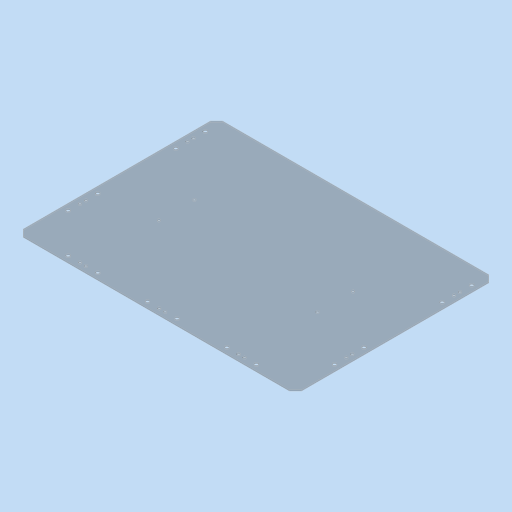
# Autodesk Inventor part: enc-SidePanel Unten 500x708
Saved by Autodesk Inventor 2023.2 (Build 272271000, 271)
## iProperties
Created: 2023-11-30
Part Number: enc-SidePanel Unten 500x708
Material: Generisch
Document SubType Name: Modeling
Designer: Nils Bade
Density: 1 g/cm^3
Appearance: PVC Verglasung
Author: Nils Bade
Autodesk Inventor part; units mm, degrees
ref_plane "YZ Plane" through (0, 0, 0) normal (1, 0, 0) x (0, 1, 0)
ref_plane "XZ Plane" through (0, 0, 0) normal (0, 1, 0) x (-1, 0, 0)
ref_plane "XY Plane" through (0, 0, 0) normal (0, 0, 1) x (1, 0, 0)
sketch "Skizze1" plane through (0, 0, 0) normal (0, 1, 0) x (-1, 0, 0)
  line L0 (0, 0) -> (-698, 0)
  line L1 (-698, 0) -> (-698, 500)
  line L2 (-698, 500) -> (0, 500)
  line L3 (0, 500) -> (0, 0)
  line L4 (-349, 0) -> (-349, 500) construction
  line L5 (0, 250) -> (-698, 250) construction
  line L6 (-150, 0) -> (-150, 500) construction
  line L7 (-548, 0) -> (-548, 500) construction
  line L8 (-698, 350) -> (0, 350) construction
  line L9 (0, 80) -> (-698, 80) construction
  line L10 (-683, 485) -> (-683, 15) construction
  line L11 (-683, 15) -> (-15, 15) construction
  line L12 (-15, 15) -> (-15, 485) construction
  line L13 (-15, 485) -> (-683, 485) construction
  line L14 (-23, 302.5) -> (-7, 302.5) construction
  line L15 (-7, 302.5) -> (-7, 397.5) construction
  line L16 (-7, 397.5) -> (-23, 397.5) construction
  line L17 (-23, 397.5) -> (-23, 302.5) construction
  line L18 (-23, 302.5) -> (-7, 397.5) construction
  line L19 (-7, 302.5) -> (-23, 397.5) construction
  line L20 (-102.5, 493) -> (-197.5, 493) construction
  line L21 (-197.5, 493) -> (-197.5, 477) construction
  line L22 (-197.5, 477) -> (-102.5, 477) construction
  line L23 (-102.5, 477) -> (-102.5, 493) construction
  line L24 (-102.5, 493) -> (-197.5, 477) construction
  line L25 (-197.5, 493) -> (-102.5, 477) construction
  line L26 (-301.5, 493) -> (-396.5, 493) construction
  line L27 (-396.5, 493) -> (-396.5, 477) construction
  line L28 (-396.5, 477) -> (-301.5, 477) construction
  line L29 (-301.5, 477) -> (-301.5, 493) construction
  line L30 (-301.5, 493) -> (-396.5, 477) construction
  line L31 (-396.5, 493) -> (-301.5, 477) construction
  circle A0 centre (-15, 342.5) radius 3.25
  circle A1 centre (-15, 313) radius 4.5
  circle A2 centre (-15, 357.5) radius 3.25
  circle A3 centre (-15, 387) radius 4.5
  circle A4 centre (-142.5, 485) radius 3.25
  circle A5 centre (-113, 485) radius 4.5
  circle A6 centre (-312, 485) radius 4.5
  circle A7 centre (-341.5, 485) radius 3.25
  circle A8 centre (-157.5, 485) radius 3.25
  circle A9 centre (-187, 485) radius 4.5
  circle A10 centre (-386, 485) radius 4.5
  circle A11 centre (-356.5, 485) radius 3.25
  circle A12 centre (-683, 342.5) radius 3.25
  circle A13 centre (-683, 313) radius 4.5
  circle A14 centre (-683, 387) radius 4.5
  circle A15 centre (-683, 357.5) radius 3.25
  circle A16 centre (-555.5, 485) radius 3.25
  circle A17 centre (-585, 485) radius 4.5
  circle A18 centre (-540.5, 485) radius 3.25
  circle A19 centre (-511, 485) radius 4.5
  circle A20 centre (-15, 43) radius 4.5
  circle A21 centre (-15, 72.5) radius 3.25
  circle A22 centre (-150, 205.5) radius 3.25
  line L32 (-138.5, 196) -> (-161.5, 196) construction
  line L33 (-161.5, 196) -> (-161.5, 304) construction
  line L34 (-161.5, 304) -> (-138.5, 304) construction
  line L35 (-138.5, 304) -> (-138.5, 196) construction
  line L36 (-138.5, 196) -> (-161.5, 304) construction
  line L37 (-161.5, 196) -> (-138.5, 304) construction
  circle A23 centre (-150, 294.5) radius 3.25
  circle A24 centre (-548, 205.5) radius 3.25
  circle A25 centre (-548, 294.5) radius 3.25
  circle A26 centre (-15, 117) radius 4.5
  circle A27 centre (-15, 87.5) radius 3.25
  circle A28 centre (-683, 43) radius 4.5
  circle A29 centre (-683, 72.5) radius 3.25
  circle A30 centre (-683, 87.5) radius 3.25
  circle A31 centre (-683, 117) radius 4.5
  point P0 (-15, 350)
  point P1 (-150, 485)
  point P2 (-349, 485)
  point P3 (-150, 250)
  dimension "d0" = 698
  dimension "d1" = 500
  dimension "d2" = 150
  dimension "d3" = 80
  dimension "d4" = 150
  dimension "d5" = 150
  dimension "d6" = 15
  dimension "d7" = 16
  dimension "d8" = 95
  dimension "d9" = 95
  dimension "d10" = 16
  dimension "d11" = 95
  dimension "d12" = 16
  dimension "d13" = 6.5
  dimension "d14" = 7.5
  dimension "d15" = 9
  dimension "d16" = 37
  dimension "d17" = 6.5
  dimension "d18" = 9
  dimension "d19" = 7.5
  dimension "d20" = 37
  dimension "d21" = 6.5
  dimension "d22" = 9
  dimension "d23" = 7.5
  dimension "d24" = 37
  dimension "d30" = 6.5
  dimension "d31" = 44.5
  dimension "d32" = 23
  dimension "d33" = 108
  dimension "d34" = 6.5
  dimension "d35" = 9
  dimension "d36" = 7.5
  dimension "d37" = 37
  constraints: 76 end point, 32 centre point, 23 symmetric about line, 21 point on line, 14 midpoint, 12 parallel, 10 perpendicular, 5 horizontal, 26 other
  measures "d0" distance of L0.start L0.end
  measures "d1" distance of L2.end L0.start
  measures "d2" distance between parallel lines of L2 L8
  measures "d3" distance between parallel lines of L0 L9
  measures "d4" distance between parallel lines of L3 L6
  measures "d5" distance between parallel lines of L1 L7
  measures "d6" distance between parallel lines of L1 L10
  measures "d7" distance of L16.end L15.end
  measures "d8" distance of L15.end L14.end
  measures "d9" distance of L22.end L21.end
  measures "d10" distance of L21.end L20.end
  measures "d11" distance of L28.end L27.end
  measures "d12" distance of L27.end L26.end
  measures "d13" diameter of A0
  measures "d14" distance from line of L8 A0.centre
  measures "d15" diameter of A1
  measures "d16" distance from line of L8 A1.centre
  measures "d17" diameter of A4
  measures "d18" diameter of A5
  measures "d19" distance from line of L6 A4.centre
  measures "d20" distance from line of L6 A5.centre
  measures "d21" diameter of A7
  measures "d22" diameter of A6
  measures "d23" distance from line of L4 A7.centre
  measures "d24" distance from line of L4 A6.centre
  measures "d30" diameter of A22
  measures "d31" distance from line of L5 A22.centre
  measures "d32" distance of L33.end L34.end
  measures "d33" distance of L32.end L33.end
  measures "d34" diameter of A21
  measures "d35" diameter of A20
  measures "d36" distance from line of L9 A21.centre
  measures "d37" distance from line of L9 A20.centre
extrude "Extrusion1" add sketch "Skizze1" along normal blind 3
chamfer "Fase1" distance 15 angle 45 4 edges at (0, 1.5, 500) (698, 1.5, 500) (698, 1.5, 0) (0, 1.5, 0)
equation "\"d5\" = d4"
equation "\"d17\" = d13"
equation "\"d18\" = d15"
equation "\"d19\" = d14"
equation "\"d20\" = d16"
equation "\"d21\" = d13"
equation "\"d22\" = d15"
equation "\"d23\" = d14"
equation "\"d24\" = d16"
equation "\"d34\" = d13"
equation "\"d35\" = d15"
equation "\"d36\" = d14"
equation "\"d37\" = d16"
